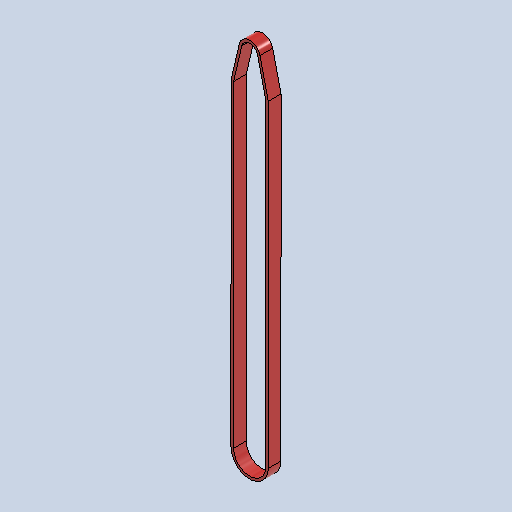
# Autodesk Inventor part: Triple Indexer band
Saved by Autodesk Inventor 2023.2 (Build 272271030, 271C)
## iProperties
Created: 2023-04-07
Part Number: Triple Indexer band
Material: Generic
Document SubType Name: Modeling
Designer: Main Account
Density: 1 g/cm^3
Appearance: Default
Author: Main Account
Autodesk Inventor part; units mm, degrees
ref_plane "YZ Plane" through (0, 0, 0) normal (1, 0, 0) x (0, 1, 0)
ref_plane "XZ Plane" through (0, 0, 0) normal (0, 1, 0) x (-1, 0, 0)
ref_plane "XY Plane" through (0, 0, 0) normal (0, 0, 1) x (1, 0, 0)
sketch "Sketch1" plane through (0, 0, 0) normal (0, 0, 1) x (1, 0, 0)
  circle A0 centre (6, 6) radius 6.35 construction
  arc A1 (-0.35, 6.0007) -> (12.35, 5.9993) centre (6, 6) ccw
  circle A2 centre (6.0155, 144.2813) radius 6.35 construction
  arc A3 (9.1061, 145.0085) -> (2.925, 145.0092) centre (6.0155, 144.2813) ccw
  line L0 (-0.336, 131.1629) -> (-0.3362, 129.9945) construction
  line L1 (12.364, 131.1615) -> (12.3638, 129.9931) construction
  line L2 (12.364, 131.1615) -> (9.1061, 145.0085)
  line L3 (2.925, 145.0092) -> (-0.336, 131.1629)
  line L4 (12.364, 131.1615) -> (12.3638, 129.9931)
  line L5 (-0.336, 131.1629) -> (-0.3362, 129.9945)
  line L6 (-0.3362, 129.9945) -> (-0.35, 6.0007)
  line L7 (12.35, 5.9993) -> (12.3638, 129.9931)
  line L8 (13.35, 129.2896) -> (13.35, 130.5741)
  line L9 (-1.35, 130.5741) -> (-1.35, 129.2896)
  line L10 (13.3638, 129.993) -> (13.364, 131.2775)
  line L11 (13.364, 131.2775) -> (10.0795, 145.2375)
  arc A4 (10.0795, 145.2375) -> (1.9516, 145.2384) centre (6.0155, 144.2813) ccw
  line L12 (1.9516, 145.2384) -> (-1.336, 131.2791)
  line L13 (-1.336, 131.2791) -> (-1.3362, 129.9946)
  line L14 (-1.3362, 129.9946) -> (-1.35, 6.0008)
  arc A5 (-1.35, 6.0008) -> (13.35, 5.9992) centre (6, 6) ccw
  line L15 (13.35, 5.9992) -> (13.3638, 129.993)
  point P0 (0, 0)
  point P1 (8.7925, 140.4734)
  point P2 (9.2272, 146.2258)
  point P3 (8.0394, 130.5099)
  point P4 (9.9436, 147.8903)
  point P5 (10.3642, 148.0002)
  point P6 (9.4208, 148.7872)
  dimension "d0" = 6.35
  dimension "d5" = 1
  constraints: 28 end point, 8 point on circle, 4 centre point, 4 tangent, 2 coincident, 2 collinear, 1 concentric, 7 other
  measures "d0" diameter of A3
  measures "d5" distance between parallel lines of L7 L15
extrude "Extrusion1" add sketch "Sketch1" along normal blind 5
body "Solid1"
